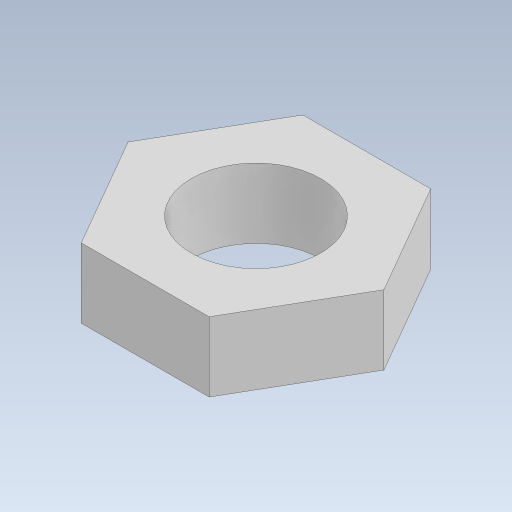
# Autodesk Inventor part: nut_thin_M4
Saved by Autodesk Inventor 2023 (Build 270158000, 158)
## iProperties
Created: 2023-05-19
Part Number: nut_thin_M4
Material: 一般
Document SubType Name: Modeling
Designer: Johnny Jou
Density: 1 g/cm^3
Appearance: 預設
Author: Johnny Jou
Autodesk Inventor part; units mm, degrees
ref_plane "YZ Plane" through (0, 0, 0) normal (1, 0, 0) x (0, 1, 0)
ref_plane "XZ Plane" through (0, 0, 0) normal (0, 1, 0) x (-1, 0, 0)
ref_plane "XY Plane" through (0, 0, 0) normal (0, 0, 1) x (1, 0, 0)
sketch "草圖1" plane through (0, 0, 0) normal (0, 1, 0) x (-1, 0, 0)
  circle A0 centre (0, 0) radius 2
  line L0 (1.9774, -3.425) -> (-1.9774, -3.425)
  line L1 (-1.9774, -3.425) -> (-3.9548, 0)
  line L2 (-3.9548, 0) -> (-1.9774, 3.425)
  line L3 (-1.9774, 3.425) -> (1.9774, 3.425)
  line L4 (1.9774, 3.425) -> (3.9548, 0)
  line L5 (3.9548, 0) -> (1.9774, -3.425)
  dimension "d0" = 4
  dimension "d1" = 6.85
  constraints: 12 end point, 2 coincident, 1 centre point, 1 horizontal, 13 other
  measures "d0" diameter of A0
  measures "d1" distance between parallel lines of L0 L3
extrude "擠出1" add sketch "草圖1" along normal blind 2.15
